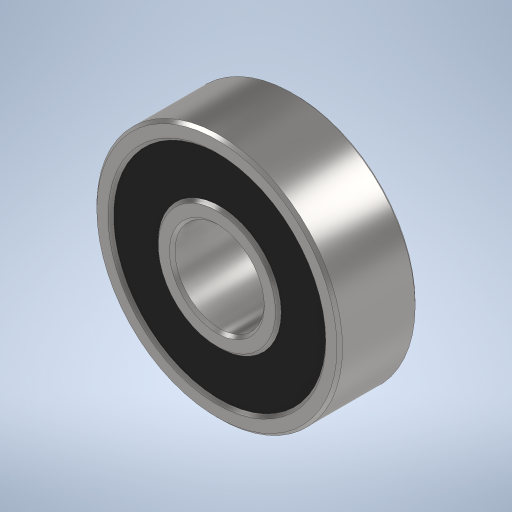
# Autodesk Inventor part: 608-2RS Bearing
Saved by Autodesk Inventor 2024 (Build 280153000, 153)
## iProperties
Created: 2024-08-10
Part Number: 608-2RS Bearing
Material: Steel, Carbon
Document SubType Name: Modeling
Designer: Ishaan
Density: 7.85 g/cm^3
Appearance: Semi-Polished
Author: Ishaan
Autodesk Inventor part; units mm, degrees
ref_plane "YZ Plane" through (0, 0, 0) normal (1, 0, 0) x (0, 1, 0)
ref_plane "XZ Plane" through (0, 0, 0) normal (0, 1, 0) x (-1, 0, 0)
ref_plane "XY Plane" through (0, 0, 0) normal (0, 0, 1) x (1, 0, 0)
sketch "Sketch1" plane through (0, 0, 0) normal (0, 0, 1) x (1, 0, 0)
  circle A0 centre (0, 0) radius 11
  circle A1 centre (0, 0) radius 4
  circle A2 centre (0, 0) radius 9.5
  circle A3 centre (0, 0) radius 5.5
  dimension "d0" = 22
  dimension "d1" = 8
  dimension "d2" = 1.5
  dimension "d3" = 1.5
  constraints: 4 centre point, 2 coincident
  measures "d0" diameter of A0
  measures "d1" diameter of A1
  measures "d2" radial gap between concentric circles of A0 A2
  measures "d3" radial gap between concentric circles of A1 A3
extrude "Extrusion1" add sketch "Sketch1" along normal mid plane 7
extrude "Extrusion2" add sketch "Sketch1" along normal mid plane 6.5 contours A2
chamfer "Chamfer1" distance 0.25 angle 45 8 edges at (-9.5, 0, 3.5) (-11, 0, 3.5) (-4, 0, -3.5) (-5.5, 0, -3.5) (-9.5, 0, -3.5) (-11, 0, -3.5) (-5.5, 0, 3.5) (-4, 0, 3.5)
body "Solid1"
